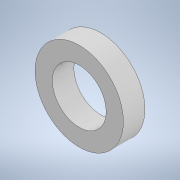
# Autodesk Inventor part: 17HS4401ShaftPlate
Saved by Autodesk Inventor 2020.2 (Build 242310000, 310)
## iProperties
Created: 2020-05-22
Part Number: 17HS4401ShaftPlate
Material: Generic
Document SubType Name: Modeling
Designer: elmar
Density: 1 g/cm^3
Appearance: Default
Author: elmar
Autodesk Inventor part; units mm, degrees
ref_plane "YZ Plane" through (0, 0, 0) normal (1, 0, 0) x (0, 1, 0)
ref_plane "XZ Plane" through (0, 0, 0) normal (0, 1, 0) x (-1, 0, 0)
ref_plane "XY Plane" through (0, 0, 0) normal (0, 0, 1) x (1, 0, 0)
sketch "Sketch1" plane through (0, 0, 0) normal (0, 0, 1) x (1, 0, 0)
  circle A0 centre (0, 0) radius 2.5
  circle A1 centre (0, 0) radius 4.1
  dimension "d0" = 8.2
  dimension "d1" = 5
  constraints: 2 centre point, 2 coincident
  measures "d0" diameter of A1
  measures "d1" diameter of A0
extrude "Extrusion1" add sketch "Sketch1" along normal blind 2
body "Solid1"
